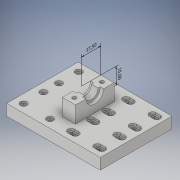
# Autodesk Inventor part: ExtruderHolder
Saved by Autodesk Inventor 2019 (Build 230136000, 136)
## iProperties
Created: 2018-06-27
Part Number: ExtruderHolder
Material: Ogólny
Document SubType Name: Modeling
Designer: Kamil
Density: 1 g/cm^3
Appearance: Domyślna
Author: Kamil
## iProperties of the stored document ExtruderHolder_Drukowanie 3D.ipt
Created: 2018-06-27
Part Number: ExtruderHolder_Drukowanie 3D
Material: Ogólny
Document SubType Name: Modeling
Designer: Kamil
Density: 1 g/cm^3
Appearance: Domyślna
Author: Kamil
Autodesk Inventor part; units mm, degrees
ref_plane "YZ Plane" through (0, 0, 0) normal (1, 0, 0) x (0, 1, 0)
ref_plane "XZ Plane" through (0, 0, 0) normal (0, 1, 0) x (-1, 0, 0)
ref_plane "XY Plane" through (0, 0, 0) normal (0, 0, 1) x (1, 0, 0)
sketch "Szkic1" plane through (0, 0, 0) normal (0, 1, 0) x (-1, 0, 0)
  circle A0 centre (34.5, 25) radius 1.75
  circle A1 centre (34.5, -25) radius 1.75
  circle A2 centre (34.5, 7) radius 1.75
  circle A3 centre (34.5, -7) radius 1.75
  line L0 (-32.5, 25) -> (-36.5, 25) construction
  line L1 (-32.5, 26.75) -> (-36.5, 26.75)
  line L2 (-36.5, 23.25) -> (-32.5, 23.25)
  arc A4 (-32.5, 23.25) -> (-32.5, 26.75) centre (-32.5, 25) ccw
  arc A5 (-36.5, 26.75) -> (-36.5, 23.25) centre (-36.5, 25) ccw
  line L3 (-42.5, 32.5) -> (42.5, 32.5)
  line L4 (42.5, 32.5) -> (42.5, -32.5)
  line L5 (42.5, -32.5) -> (-42.5, -32.5)
  line L6 (-42.5, -32.5) -> (-42.5, 32.5)
  line L7 (-42.5, 32.5) -> (42.5, -32.5) construction
  line L8 (42.5, 32.5) -> (-42.5, -32.5) construction
  line L9 (-36.5, 7) -> (-32.5, 7) construction
  line L10 (-36.5, 5.25) -> (-32.5, 5.25)
  line L11 (-32.5, 8.75) -> (-36.5, 8.75)
  arc A6 (-36.5, 8.75) -> (-36.5, 5.25) centre (-36.5, 7) ccw
  arc A7 (-32.5, 5.25) -> (-32.5, 8.75) centre (-32.5, 7) ccw
  line L12 (-36.5, -7) -> (-32.5, -7) construction
  line L13 (-36.5, -8.75) -> (-32.5, -8.75)
  line L14 (-32.5, -5.25) -> (-36.5, -5.25)
  arc A8 (-36.5, -5.25) -> (-36.5, -8.75) centre (-36.5, -7) ccw
  arc A9 (-32.5, -8.75) -> (-32.5, -5.25) centre (-32.5, -7) ccw
  circle A10 centre (10.5, 25) radius 1.75
  circle A11 centre (10.5, 7) radius 1.75
  circle A12 centre (10.5, -7) radius 1.75
  circle A13 centre (10.5, -25) radius 1.75
  line L15 (-36.5, -25) -> (-32.5, -25) construction
  line L16 (-36.5, -26.75) -> (-32.5, -26.75)
  line L17 (-32.5, -23.25) -> (-36.5, -23.25)
  arc A14 (-36.5, -23.25) -> (-36.5, -26.75) centre (-36.5, -25) ccw
  arc A15 (-32.5, -26.75) -> (-32.5, -23.25) centre (-32.5, -25) ccw
  line L18 (-34.5, -25) -> (-30.5, -25) construction
  line L19 (-12.5, -7) -> (-8.5, -7) construction
  line L20 (-12.5, -8.75) -> (-8.5, -8.75)
  line L21 (-8.5, -5.25) -> (-12.5, -5.25)
  arc A16 (-12.5, -5.25) -> (-12.5, -8.75) centre (-12.5, -7) ccw
  arc A17 (-8.5, -8.75) -> (-8.5, -5.25) centre (-8.5, -7) ccw
  line L22 (-12.5, -25) -> (-8.5, -25) construction
  line L23 (-12.5, -26.75) -> (-8.5, -26.75)
  line L24 (-8.5, -23.25) -> (-12.5, -23.25)
  arc A18 (-12.5, -23.25) -> (-12.5, -26.75) centre (-12.5, -25) ccw
  arc A19 (-8.5, -26.75) -> (-8.5, -23.25) centre (-8.5, -25) ccw
  line L25 (-12.5, 7) -> (-8.5, 7) construction
  line L26 (-12.5, 5.25) -> (-8.5, 5.25)
  line L27 (-8.5, 8.75) -> (-12.5, 8.75)
  arc A20 (-12.5, 8.75) -> (-12.5, 5.25) centre (-12.5, 7) ccw
  arc A21 (-8.5, 5.25) -> (-8.5, 8.75) centre (-8.5, 7) ccw
  line L28 (-10.5, 7) -> (-6.5, 7) construction
  line L29 (-12.5, 25) -> (-8.5, 25) construction
  line L30 (-12.5, 23.25) -> (-8.5, 23.25)
  line L31 (-8.5, 26.75) -> (-12.5, 26.75)
  arc A22 (-12.5, 26.75) -> (-12.5, 23.25) centre (-12.5, 25) ccw
  arc A23 (-8.5, 23.25) -> (-8.5, 26.75) centre (-8.5, 25) ccw
  point P0 (0, 0)
  point P1 (-34.5, 25)
  point P2 (-34.5, 7)
  point P3 (-34.5, -7)
  point P4 (-10.5, -7)
  point P5 (-10.5, -25)
  point P6 (-10.5, 25)
  dimension "d2" = 3.5
  dimension "d3" = 3.5
  dimension "d7" = 3.5
  dimension "d8" = 3.5
  dimension "d9" = 2
  dimension "d10" = 3.5
  dimension "d11" = 85
  dimension "d12" = 65
  dimension "d13" = 2
  dimension "d14" = 3.5
  dimension "d15" = 2
  dimension "d16" = 3.5
  dimension "d19" = 3.5
  dimension "d20" = 3.5
  dimension "d21" = 3.5
  dimension "d22" = 3.5
  dimension "d23" = 2
  dimension "d24" = 0
  dimension "d25" = 3.5
  dimension "d26" = 2
  dimension "d27" = 3.5
  dimension "d28" = 2
  dimension "d29" = 3.5
  dimension "d30" = 2
  dimension "d31" = 0
  dimension "d32" = 3.5
  dimension "d33" = 2
  dimension "d34" = 3.5
  constraints: 80 end point, 32 point on circle, 32 tangent, 24 centre point, 14 parallel, 10 midpoint, 6 horizontal, 2 collinear, 1 perpendicular
  measures "d2" diameter of A0
  measures "d3" diameter of A1
  measures "d7" diameter of A2
  measures "d8" diameter of A3
  measures "d9" distance of point (-34.5, 25) L0.end
  measures "d10" diameter of A5
  measures "d11" distance of L4.end L5.end
  measures "d12" distance of L3.end L4.end
  measures "d13" distance of point (-34.5, 7) L9.end
  measures "d14" diameter of A7
  measures "d15" distance of point (-34.5, -7) L12.end
  measures "d16" diameter of A9
  measures "d19" diameter of A10
  measures "d20" diameter of A11
  measures "d21" diameter of A12
  measures "d22" diameter of A13
  measures "d23" distance of L18.start L15.end
  measures "d24" distance between parallel lines of L15 L18
  measures "d25" diameter of A15
  measures "d26" distance of point (-10.5, -7) L19.end
  measures "d27" diameter of A17
  measures "d28" distance of point (-10.5, -25) L22.end
  measures "d29" diameter of A19
  measures "d30" distance of L28.start L25.end
  measures "d31" distance between parallel lines of L25 L28
  measures "d32" diameter of A21
  measures "d33" distance of point (-10.5, 25) L29.end
  measures "d34" diameter of A23
extrude "Wyciągnięcie proste1" add sketch "Szkic1" along normal blind 10
sketch "Szkic2" plane through (0, 10, 0) normal (0, 1, 0) x (1, 0, 0)
  circle A0 centre (-34.5, -25) radius 3
  circle A1 centre (-34.5, -7) radius 3
  circle A2 centre (-34.5, 7) radius 3
  circle A3 centre (-34.5, 25) radius 3
  circle A4 centre (-10.5, -25) radius 3
  circle A5 centre (-10.5, -7) radius 3
  circle A6 centre (-10.5, 7) radius 3
  circle A7 centre (-10.5, 25) radius 3
  line L0 (8.5, -25) -> (12.5, -25) construction
  line L1 (8.5, -28) -> (12.5, -28)
  line L2 (12.5, -22) -> (8.5, -22)
  arc A8 (8.5, -22) -> (8.5, -28) centre (8.5, -25) ccw
  arc A9 (12.5, -28) -> (12.5, -22) centre (12.5, -25) ccw
  line L3 (8.5, -7) -> (12.5, -7) construction
  line L4 (8.5, -10) -> (12.5, -10)
  line L5 (12.5, -4) -> (8.5, -4)
  arc A10 (8.5, -4) -> (8.5, -10) centre (8.5, -7) ccw
  arc A11 (12.5, -10) -> (12.5, -4) centre (12.5, -7) ccw
  line L6 (8.5, 7) -> (12.5, 7) construction
  line L7 (8.5, 4) -> (12.5, 4)
  line L8 (12.5, 10) -> (8.5, 10)
  arc A12 (8.5, 10) -> (8.5, 4) centre (8.5, 7) ccw
  arc A13 (12.5, 4) -> (12.5, 10) centre (12.5, 7) ccw
  line L9 (8.5, 25) -> (12.5, 25) construction
  line L10 (8.5, 22) -> (12.5, 22)
  line L11 (12.5, 28) -> (8.5, 28)
  arc A14 (8.5, 28) -> (8.5, 22) centre (8.5, 25) ccw
  arc A15 (12.5, 22) -> (12.5, 28) centre (12.5, 25) ccw
  line L12 (32.5, -25) -> (36.5, -25) construction
  line L13 (32.5, -28) -> (36.5, -28)
  line L14 (36.5, -22) -> (32.5, -22)
  arc A16 (32.5, -22) -> (32.5, -28) centre (32.5, -25) ccw
  arc A17 (36.5, -28) -> (36.5, -22) centre (36.5, -25) ccw
  line L15 (32.5, -7) -> (36.5, -7) construction
  line L16 (32.5, -10) -> (36.5, -10)
  line L17 (36.5, -4) -> (32.5, -4)
  arc A18 (32.5, -4) -> (32.5, -10) centre (32.5, -7) ccw
  arc A19 (36.5, -10) -> (36.5, -4) centre (36.5, -7) ccw
  line L18 (32.5, 7) -> (36.5, 7) construction
  line L19 (32.5, 4) -> (36.5, 4)
  line L20 (36.5, 10) -> (32.5, 10)
  arc A20 (32.5, 10) -> (32.5, 4) centre (32.5, 7) ccw
  arc A21 (36.5, 4) -> (36.5, 10) centre (36.5, 7) ccw
  line L21 (32.5, 25) -> (36.5, 25) construction
  line L22 (32.5, 22) -> (36.5, 22)
  line L23 (36.5, 28) -> (32.5, 28)
  arc A22 (32.5, 28) -> (32.5, 22) centre (32.5, 25) ccw
  arc A23 (36.5, 22) -> (36.5, 28) centre (36.5, 25) ccw
  point P0 (0, 0)
  point P1 (10.5, -25)
  point P2 (10.5, -7)
  point P3 (10.5, 7)
  point P4 (10.5, 25)
  point P5 (34.5, -25)
  point P6 (34.5, -7)
  point P7 (34.5, 7)
  point P8 (34.5, 25)
  dimension "d37" = 6
  dimension "d38" = 6
  dimension "d39" = 6
  dimension "d40" = 6
  dimension "d41" = 6
  dimension "d42" = 6
  dimension "d43" = 6
  dimension "d44" = 6
  dimension "d45" = 2
  dimension "d46" = 6
  dimension "d47" = 2
  dimension "d48" = 6
  dimension "d49" = 2
  dimension "d50" = 6
  dimension "d51" = 2
  dimension "d52" = 6
  dimension "d53" = 2
  dimension "d54" = 6
  dimension "d55" = 2
  dimension "d56" = 6
  dimension "d57" = 2
  dimension "d58" = 6
  dimension "d59" = 2
  dimension "d60" = 6
  constraints: 64 end point, 32 point on circle, 32 tangent, 24 centre point, 11 parallel, 8 midpoint, 8 point on line, 1 horizontal
  measures "d37" diameter of A0
  measures "d38" diameter of A1
  measures "d39" diameter of A2
  measures "d40" diameter of A3
  measures "d41" diameter of A4
  measures "d42" diameter of A5
  measures "d43" diameter of A6
  measures "d44" diameter of A7
  measures "d45" distance of point (10.5, -25) L0.end
  measures "d46" diameter of A9
  measures "d47" distance of point (10.5, -7) L3.end
  measures "d48" diameter of A11
  measures "d49" distance of point (10.5, 7) L6.end
  measures "d50" diameter of A13
  measures "d51" distance of point (10.5, 25) L9.end
  measures "d52" diameter of A15
  measures "d53" distance of point (34.5, -25) L12.end
  measures "d54" diameter of A17
  measures "d55" distance of point (34.5, -7) L15.end
  measures "d56" diameter of A19
  measures "d57" distance of point (34.5, 7) L18.end
  measures "d58" diameter of A21
  measures "d59" distance of point (34.5, 25) L21.end
  measures "d60" diameter of A23
extrude "Wyciągnięcie proste2" cut sketch "Szkic2" against normal blind 2
sketch "Szkic5" plane through (0, 10, 0) normal (0, 1, 0) x (1, 0, 0)
  line L0 (5, -17.5) -> (-7, -17.5)
  line L1 (-7, -17.5) -> (-7, 17.5)
  line L2 (-7, 17.5) -> (5, 17.5)
  line L3 (5, 17.5) -> (5, -17.5)
  line L4 (5, -17.5) -> (-7, 17.5) construction
  line L5 (-7, -17.5) -> (5, 17.5) construction
  point P0 (0, 0)
  point P1 (-1, 0)
  dimension "d69" = 12
  dimension "d70" = 35
  constraints: 12 end point, 2 midpoint, 2 parallel, 1 horizontal, 1 perpendicular
  measures "d69" distance of L1.end L2.end
  measures "d70" distance of L0.end L1.end
extrude "Wyciągnięcie proste4" add sketch "Szkic5" along normal blind 15
sketch "Szkic6" plane through (-7, 10, -17.5) normal (-1, 0, 0) x (0, 0, 1)
  arc A0 (11.5, 15) -> (23.5, 15) centre (17.5, 15) ccw
  line L0 (25.5, 15) -> (23.5, 15)
  line L1 (23.5, 15) -> (11.5, 15)
  arc A1 (9.5, 15) -> (25.5, 15) centre (17.5, 15) ccw
  line L2 (11.5, 15) -> (9.5, 15)
  point P0 (17.5, -10)
  dimension "d73" = 12
  constraints: 6 end point, 4 point on circle, 3 horizontal, 2 centre point, 1 coincident
  measures "d73" diameter of A0
sketch "Szkic7" plane through (5, 10, 17.5) normal (1, 0, 0) x (0, 0, -1)
  line L0 (9.5, 15) -> (25.5, 15)
  arc A0 (9.5, 15) -> (25.5, 15) centre (17.5, 15) ccw
  point P0 (17.5, -10)
  constraints: 2 end point, 2 point on circle, 1 centre point, 1 horizontal
extrude "Wyciągnięcie proste5" cut sketch "Szkic6" against normal blind 3 contours A0 L0 A1 L2
extrude "Wyciągnięcie proste6" cut sketch "Szkic7" against normal blind 3
sketch "Szkic8" plane through (-7, 25, 0) normal (-1, 0, 0) x (0, 0, 1)
  line L0 (6, 0) -> (-6, 0)
  arc A0 (-6, 0) -> (6, 0) centre (0, 0) ccw
  point P0 (0, -25)
  constraints: 2 end point, 2 point on circle, 1 centre point, 1 horizontal
extrude "Wyciągnięcie proste7" cut sketch "Szkic8" against normal blind 9
sketch "Szkic9" plane through (0, 25, 0) normal (0, 1, 0) x (1, 0, 0)
  circle A0 centre (-1, 12.5) radius 1.75
  circle A1 centre (-1, -12.5) radius 1.75
  point P0 (0, 0)
  dimension "d83" = 3.5
  dimension "d84" = 3.5
  constraints: 2 centre point
  measures "d83" diameter of A0
  measures "d84" diameter of A1
sketch "Szkic10" plane through (-7, 10, -17.5) normal (-1, 0, 0) x (0, 0, 1)
  line L0 (8, 6.5) -> (2, 6.5)
  line L1 (2, 6.5) -> (2, 3.5)
  line L2 (2, 3.5) -> (8, 3.5)
  line L3 (8, 3.5) -> (8, 6.5)
  line L4 (8, 6.5) -> (2, 3.5) construction
  line L5 (2, 6.5) -> (8, 3.5) construction
  line L6 (33, 6.5) -> (27, 6.5)
  line L7 (27, 6.5) -> (27, 3.5)
  line L8 (27, 3.5) -> (33, 3.5)
  line L9 (33, 3.5) -> (33, 6.5)
  line L10 (33, 6.5) -> (27, 3.5) construction
  line L11 (27, 6.5) -> (33, 3.5) construction
  point P0 (17.5, -10)
  point P1 (5, 5)
  point P2 (30, 5)
  dimension "d91" = 6
  dimension "d92" = 3
  dimension "d93" = 6
  dimension "d94" = 3
  constraints: 24 end point, 4 midpoint, 4 parallel, 2 horizontal, 2 perpendicular
  measures "d91" distance of L2.end L1.end
  measures "d92" distance of L1.end L0.end
  measures "d93" distance of L8.end L7.end
  measures "d94" distance of L7.end L6.end
extrude "Wyciągnięcie proste9" cut sketch "Szkic10" against normal blind 9.5
extrude "Wyciągnięcie proste10" cut sketch "Szkic9" against normal blind 25
